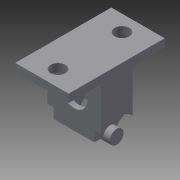
# Autodesk Inventor part: chain_end_2020-back
Saved by Autodesk Inventor 2014 (Build 180170000, 170)
## iProperties
Created: 2016-05-16
Part Number: chain_end_2020-back
Material: Generic
Document SubType Name: Modeling
Designer: 101767
Density: 1 g/cm^3
Appearance: Default
Author: 101767
Autodesk Inventor part; units mm, degrees
ref_plane "YZ Plane" through (0, 0, 0) normal (1, 0, 0) x (0, 1, 0)
sketch "Sketch1" plane through (0, 0, 0) normal (0, 0, 1) x (1, 0, 0)
  line L0 (0, 0) -> (15.2, 0)
  line L1 (15.2, 0) -> (15.2, 12)
  line L2 (15.2, 12) -> (0, 12)
  line L3 (0, 12) -> (0, 0)
  line L4 (1.6, 10) -> (13.6, 10)
  line L5 (13.6, 10) -> (13.6, 2)
  line L6 (13.6, 2) -> (1.6, 2)
  line L7 (1.6, 2) -> (1.6, 10)
  dimension "d0" = 15.2
  dimension "d1" = 12
  dimension "d2" = 1.6
  dimension "d3" = 2
  dimension "d4" = 2
  dimension "d5" = 1.6
  constraints: 16 end point, 4 parallel, 2 horizontal, 2 perpendicular
  measures "d0" distance of L1.end L2.end
  measures "d1" distance of L0.end L1.end
  measures "d2" distance between parallel lines of L3 L7
  measures "d3" distance between parallel lines of L2 L4
  measures "d4" distance between parallel lines of L0 L6
  measures "d5" distance between parallel lines of L1 L5
extrude "Extrusion1" add sketch "Sketch1" along normal blind 20
sketch "Sketch2" plane through (0, 0, 0) normal (1, 0, 0) x (0, 1, 0)
  line L0 (0, 0) -> (12, 0) construction
  line L1 (6, 13.0663) -> (6, -2.0093) construction
  line L2 (0, 0) -> (0, 20) construction
  line L3 (12, 0) -> (12, 20) construction
  line L4 (6, 0) -> (12, 3.8224)
  line L5 (12, 3.8224) -> (12, 0)
  line L6 (12, 0) -> (6, 0)
  dimension "d8" = 12
  dimension "d9" = 6
  dimension "d10" = 32.5
  constraints: 8 end point, 2 collinear, 2 point on line, 1 midpoint, 1 perpendicular
  measures "d8" distance of L0.start L0.end
  measures "d9" distance between parallel lines of L2 L1
  measures "d10" angle of L0 L4
extrude "Extrusion2" cut sketch "Sketch2" along normal through all
sketch "Sketch4" plane through (1.6, 2, 20) normal (1, 0, 0) x (0, 0, -1)
  circle A0 centre (20, 4) radius 2.6
  point P0 (20, -2)
  dimension "d14" = 5.2
  constraints: 1 centre point, 1 coincident
  measures "d14" diameter of A0
extrude "Extrusion3" add sketch "Sketch4" against normal blind 4
sketch "Sketch5" plane through (0, 0, 20) normal (-1, 0, 0) x (0, 0, 1)
  line L0 (-20, 0) -> (0, 0) construction
  line L1 (0, 12) -> (0, 0) construction
  line L2 (-16.1776, 12) -> (0, 12) construction
  arc A0 (-16.1776, 0) -> (-16.1776, 12) centre (-21.4691, 6) ccw
  line L3 (-16.1776, 12) -> (0, 12)
  line L4 (0, 0) -> (-16.1776, 0)
  line L5 (0, 0) -> (0, 12)
  dimension "d17" = 8
  constraints: 6 end point, 3 collinear, 2 point on circle, 1 centre point, 1 point on line, 1 vertical alignment
  measures "d17" radius of A0
extrude "Extrusion4" add sketch "Sketch5" along normal blind 2.4
ref_plane "Work Plane2" through (7.6, 2, 20) normal (1, 0, 0) x (0, 0, -1)
mirror "Mirror1" about plane through (7.6, 2, 20) normal (1, 0, 0) of "Extrusion3", "Extrusion4"
sketch "Sketch6" plane through (0, 0, 20) normal (0, 0, 1) x (1, 0, 0)
  line L0 (17.6, 0) -> (17.6, 12) construction
  line L1 (-2.4, 12) -> (17.6, 12) construction
  line L2 (-2.4, 0) -> (-2.4, 12) construction
  line L3 (-2.4, 0) -> (-2.4, 24)
  line L4 (-2.4, 24) -> (17.6, 24)
  line L5 (17.6, 24) -> (17.6, 0)
  line L6 (-2.4, 0) -> (-2.4, -12)
  line L7 (-2.4, -12) -> (17.6, -12)
  line L8 (17.6, -12) -> (17.6, 0)
  point P0 (0, 0)
  dimension "d21" = 12
  dimension "d22" = 12
  constraints: 12 end point, 2 collinear, 2 perpendicular, 1 parallel, 1 point on line
  measures "d21" distance between parallel lines of L1 L4
  measures "d22" distance of L2.start L6.end
extrude "Extrusion5" add sketch "Sketch6" along normal blind 3
sketch "Sketch7" plane through (0, 0, 0) normal (0, -1, 0) x (1, 0, 0)
  line L0 (17.6, 20) -> (-2.4, 20) construction
  line L1 (0, 0) -> (0, 3.8224) construction
  line L2 (7.6, 20) -> (7.6, -5.3429) construction
  circle A0 centre (7.6, 12.3224) radius 5
  line L3 (15.2, 3.8224) -> (0, 3.8224) construction
  dimension "d25" = 10
  dimension "d26" = 8.5
  constraints: 2 end point, 1 centre point, 1 midpoint, 1 parallel, 1 point on line
  measures "d25" diameter of A0
  measures "d26" distance from line of A0.centre L3
extrude "Extrusion6" cut sketch "Sketch7" against normal through all
sketch "Sketch8" plane through (0, 0, 20) normal (0, 0, -1) x (-1, 0, 0)
  line L0 (-17.6, -12) -> (2.4, -12) construction
  line L1 (2.4, -12) -> (2.4, 0) construction
  line L2 (-7.6, -12) -> (-7.6, 4.0518) construction
  circle A0 centre (-7.6, -6) radius 2.75
  point P0 (-17.6, 0)
  point P1 (0, 0)
  dimension "d29" = 12
  dimension "d30" = 6
  dimension "d31" = 5.5
  constraints: 2 end point, 1 centre point, 1 midpoint, 1 parallel, 1 point on line
  measures "d29" distance of point (-17.6, 0) L0.start
  measures "d30" distance from line of L0 A0.centre
  measures "d31" diameter of A0
extrude "Extrusion7" cut sketch "Sketch8" against normal through all
ref_plane "Work Plane3" through (0, 6, 0) normal (0, -1, 0) x (1, 0, 0)
mirror "Mirror2" about plane through (0, 6, 0) normal (0, -1, 0) of "Extrusion7"
fillet "Fillet1" radius 2 4 edges at (14.4, 8.1928, 1.397) (0.8, 8.1928, 1.397) (14.4, 3.4, 0) (0.8, 3.4, 0)
equation "\"d9\" = 0.5 * d8"
equation "\"d22\" = d21"
equation "\"d30\" = 0.5 * d29"
body "Solid1"
